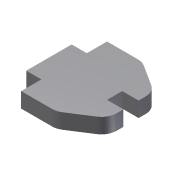
# Autodesk Inventor part: OpenROV_Dev_EChassis_Servo_Plate_Brace
Saved by Autodesk Inventor 2012 (Build 160160000, 160)
## iProperties
Created: 2012-08-07
Part Number: OpenROV_Dev_EChassis_Servo_Plate_Brace
Material: Default
Document SubType Name: Modeling
Designer: user
Density: 1 g/cm^3
Author: user
Autodesk Inventor part; units mm, degrees
ref_plane "YZ Plane" through (0, 0, 0) normal (1, 0, 0) x (0, 1, 0)
ref_plane "XZ Plane" through (0, 0, 0) normal (0, 1, 0) x (-1, 0, 0)
ref_plane "XY Plane" through (0, 0, 0) normal (0, 0, 1) x (1, 0, 0)
sketch "Sketch1" plane through (0, 0, 0) normal (0, 0, 1) x (1, 0, 0)
  line L0 (6.1221, 8.5) -> (0, 8.5)
  line L1 (0, 8.5) -> (0, 4.5)
  line L2 (0, 4.5) -> (-3, 4.5)
  line L3 (-3, 4.5) -> (-3, -4.5)
  line L4 (11.8667, -5.385) -> (7.7394, -8.0267)
  line L5 (6.1221, -8.5) -> (0, -8.5)
  line L6 (0, -8.5) -> (0, -4.5)
  line L7 (0, -4.5) -> (-3, -4.5)
  line L8 (10, 1.5) -> (10, -1.5)
  line L9 (10, -1.5) -> (13.2494, -1.5)
  line L10 (10, 1.5) -> (13.2494, 1.5)
  line L11 (13.2494, 1.5) -> (13.2494, 2.8583)
  line L12 (13.2494, -1.5) -> (13.2494, -2.8583)
  line L13 (11.8667, 5.385) -> (7.7394, 8.0267)
  arc A0 (7.7394, 8.0267) -> (6.1221, 8.5) centre (6.1221, 5.5) ccw
  arc A1 (13.2494, 2.8583) -> (11.8667, 5.385) centre (10.2494, 2.8583) ccw
  arc A2 (11.8667, -5.385) -> (13.2494, -2.8583) centre (10.2494, -2.8583) ccw
  arc A3 (6.1221, -8.5) -> (7.7394, -8.0267) centre (6.1221, -5.5) ccw
  point P0 (7, 8.5)
  point P1 (7, -8.5)
  point P2 (13.2494, 4.5)
  point P3 (13.2494, -4.5)
  point P4 (0, 0)
  dimension "d13" = 3
  dimension "d26" = 7
  dimension "d27" = 9
  dimension "d28" = 4
  dimension "d29" = 4
  dimension "d30" = 7
  dimension "d33" = 4.5
  dimension "d34" = 3
  dimension "d35" = 1.5
  dimension "d36" = 3
  dimension "d37" = 3
  dimension "d38" = 3
  dimension "d39" = 3
  constraints: 28 end point, 8 point on circle, 8 point on line, 8 tangent, 4 centre point, 4 perpendicular, 3 equal radius, 3 parallel, 1 collinear
  measures "d13" distance between parallel lines of L3 L1
  measures "d26" distance of point (7, 8.5) L0.end
  measures "d27" distance of L2.end L3.end
  measures "d28" distance of L0.end L1.end
  measures "d29" distance between parallel lines of L5 L7
  measures "d30" distance of point (7, -8.5) L5.end
  measures "d33" distance from line of point (0, 0) L2
  measures "d34" distance from line of point (0, 0) L3
  measures "d35" distance from line of point (0, 0) L10
  measures "d36" distance of L10.end point (13.249, 4.5)
  measures "d37" distance of L9.end point (13.249, -4.5)
  measures "d38" distance of L8.start L8.end
  measures "d39" radius of A0
extrude "Extrusion1" add sketch "Sketch1" along normal blind 3
body "Solid1"
